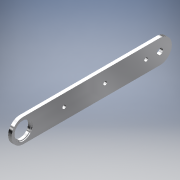
# Autodesk Inventor part: Bearing Holder
Saved by Autodesk Inventor 2019.4 (Build 234330000, 330)
## iProperties
Created: 2020-01-03
Part Number: Bearing Holder
Material: Aluminum 6061
Document SubType Name: Modeling
Designer: Mark
Mass: 100.007 g
Surface Area: 182.234 cm^2
Volume: 37.0395 cm^3
Density: 2.7 g/cm^3
Appearance: Aluminum - Flat
Author: Mark
Autodesk Inventor part; units mm, degrees
ref_plane "YZ Plane" through (0, 0, 0) normal (1, 0, 0) x (0, 1, 0)
ref_plane "XZ Plane" through (0, 0, 0) normal (0, 1, 0) x (-1, 0, 0)
ref_plane "XY Plane" through (0, 0, 0) normal (0, 0, 1) x (1, 0, 0)
sketch "Sketch1" plane through (0, 0, 0) normal (1, 0, 0) x (0, 1, 0)
  circle A0 centre (0, 0) radius 12
  circle A1 centre (0, 0) radius 17.5
  line L0 (0, 0) -> (0, -201.7) construction
  line L1 (-17.5, 0) -> (-17.5, -201.7)
  line L2 (17.5, -201.7) -> (17.5, 0)
  arc A2 (17.5, 0) -> (-17.5, 0) centre (0, 0) ccw
  arc A3 (-17.5, -201.7) -> (17.5, -201.7) centre (0, -201.7) ccw
  line L3 (0, 0) -> (201.7, 0) construction
  circle A4 centre (0, -60.425) radius 2.75
  circle A5 centre (0, -120.85) radius 2.75
  circle A6 centre (0, -181.275) radius 2.75
  circle A7 centre (0, -201.7) radius 4.5
  point P0 (0, -100.85)
  dimension "d0" = 24
  dimension "d1" = 35
  dimension "d7" = 201.7
  dimension "d8" = 90
  dimension "d9" = 35
  dimension "d13" = 5.5
  dimension "d14" = 60.425
  dimension "d15" = 17.5
  dimension "d18" = 60.425
  dimension "d23" = 9
  constraints: 10 end point, 8 centre point, 4 point on circle, 4 tangent, 3 coincident, 2 vertical, 1 horizontal, 1 midpoint, 1 parallel, 1 perpendicular, 4 other
  measures "d0" diameter of A0
  measures "d1" diameter of A1
  measures "d7" distance of L0.start L0.end
  measures "d8" angle of L0 L3
  measures "d9" diameter of A3
  measures "d13" diameter of A4
  measures "d14" distance of L0.start A4.centre
  measures "d15" distance from line of L1 A4.centre
  measures "d18" distance of A4.centre A5.centre
  measures "d23" diameter of A7
extrude "Extrusion1" add sketch "Sketch1" along normal blind 5
sketch "Sketch2" plane through (5, 0, 0) normal (1, 0, 0) x (0, 0, -1)
  circle A0 centre (0, 0) radius 13.5
  dimension "d4" = 27
  constraints: 1 centre point, 1 coincident
  measures "d4" diameter of A0
extrude "Extrusion2" cut sketch "Sketch2" against normal blind 1.1
body "Solid1"
